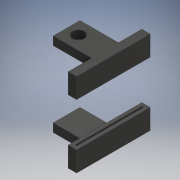
# Autodesk Inventor part: learnbotAgarreCamara
Saved by Autodesk Inventor 2017 (Build 210142000, 142)
## iProperties
Part Number: learnbotAgarreCamara
Material: Genérico
Document SubType Name: Modeling
Designer: rober
Density: 1 g/cm^3
Appearance: Valor por defecto
Author: rober
Autodesk Inventor part; units mm, degrees
ref_plane "YZ Plane" through (0, 0, 0) normal (1, 0, 0) x (0, 1, 0)
ref_plane "XZ Plane" through (0, 0, 0) normal (0, 1, 0) x (-1, 0, 0)
ref_plane "XY Plane" through (0, 0, 0) normal (0, 0, 1) x (1, 0, 0)
sketch "Boceto8" plane through (0, 0, 0) normal (0, 0, 1) x (1, 0, 0)
  line L0 (-2.8, 3) -> (-0.5, 3)
  line L1 (-0.5, 1.4) -> (-2.8, 1.4)
  line L2 (-2.8, 3) -> (-2.8, 1.4)
  line L3 (0, 3) -> (0, 0)
  line L4 (0, 0) -> (-0.5, 0)
  line L5 (-0.5, 0) -> (-0.5, 1.4)
  line L6 (0, 3) -> (0, 4.4)
  line L7 (0, 4.4) -> (-0.5, 4.4)
  line L8 (-0.5, 4.4) -> (-0.5, 3)
  constraints: 18 end point
extrude "Extrusión8" add sketch "Boceto8" along normal blind 0.5
sketch "Boceto9" plane through (0, 0, 0.5) normal (0, 0, 1) x (1, 0, 0)
  line L0 (-0.5, 3) -> (-2.8, 3) projected
  line L1 (-2.8, 3) -> (-2.8, 1.4) projected
  line L2 (-2.8, 1.4) -> (-0.5, 1.4) projected
  line L3 (-0.5, 1.4) -> (-0.5, 0) projected
  line L4 (-0.5, 0) -> (0, 0) projected
  line L5 (0, 0) -> (0, 4.4) projected
  line L6 (0, 4.4) -> (-0.5, 4.4) projected
  line L7 (-0.5, 4.4) -> (-0.5, 3) projected
  line L8 (0, 4.4) -> (0, 0) projected
  line L9 (-0.5, 4.4) -> (0, 4.4)
  line L10 (0, 4.4) -> (0, 0)
  line L11 (0, 0) -> (-0.5, 0)
  line L12 (-0.5, 0) -> (-0.5, 4.4)
  constraints: 8 end point, 2 parallel, 1 horizontal, 1 perpendicular
extrude "Extrusión9" add sketch "Boceto9" along normal blind 0.7 contours L7 L6 L5 L4 L3 L12
sketch "Boceto10" plane through (0, 0, 0) normal (0, 0, -1) x (-1, 0, 0)
  line L0 (2.8, 3) -> (0.5, 3)
  line L1 (0.5, 3) -> (0.5, 4.4)
  line L2 (0.5, 4.4) -> (0, 4.4)
  line L3 (0, 4.4) -> (0, 0)
  line L4 (0, 0) -> (0.5, 0)
  line L5 (0.5, 0) -> (0.5, 1.4)
  line L6 (0.5, 1.4) -> (2.8, 1.4)
  line L7 (2.8, 1.4) -> (2.8, 3)
  arc A0 (1.893104, 1.910428) -> (1.925936, 2.512803) centre (2.122635, 2.2) ccw
  line L8 (0.685113, 2.000554) -> (1.893104, 1.910428)
  line L9 (0.681802, 2.399171) -> (1.925936, 2.512803)
  arc A1 (0.681802, 2.399171) -> (0.685113, 2.000554) centre (0.699993, 2.2) ccw
  line L10 (2.8, 1.4) -> (0.499993, 1.4)
  line L11 (0.499993, 3) -> (2.8, 3)
  line L12 (2.8, 1.4) -> (2.8, 3)
  line L13 (-0.000007, 1.4) -> (-0.000007, 4.4)
  line L14 (-0.000007, 4.4) -> (0.499993, 4.4)
  line L15 (0.499993, 4.4) -> (0.499993, 3)
  line L16 (-0.000007, 1.4) -> (-0.000007, 0)
  line L17 (-0.000007, 0) -> (0.499993, 0)
  line L18 (0.499993, 0) -> (0.499993, 1.4)
  line L19 (0.299993, 1.4) -> (0.299993, 4.2)
  line L20 (0.299993, 4.2) -> (0.199993, 4.2)
  line L21 (0.199993, 4.2) -> (0.199993, 1.4)
  line L22 (0.299993, 1.4) -> (0.299993, 0.2)
  line L23 (0.299993, 0.2) -> (0.199993, 0.2)
  line L24 (0.199993, 0.2) -> (0.199993, 1.4)
  line L25 (0.499993, 1.4) -> (0.499993, 3)
  constraints: 36 end point, 4 point on circle, 2 centre point
sketch "Boceto10 outline for Extrusión10" plane through (0, 0, 0) normal (0, 0, -1) x (-1, 0, 0)
  line L0 (0.685113, 2.000554) -> (1.893104, 1.910428)
  arc A0 (0.681802, 2.399171) -> (0.685113, 2.000554) centre (0.699993, 2.2) ccw
  line L1 (1.925936, 2.512803) -> (0.681802, 2.399171)
  arc A1 (1.893104, 1.910428) -> (1.925936, 2.512803) centre (2.122635, 2.2) ccw
extrude "Extrusión10" cut sketch "Boceto10 outline for Extrusión10" against normal blind 0.25
sketch "Boceto11" plane through (0, 0, 1.2) normal (0, 0, 1) x (1, 0, 0)
  line L0 (0, 0) -> (0, 4.4)
  line L1 (0, 4.4) -> (-0.5, 4.4)
  line L2 (-0.5, 4.4) -> (-0.5, 0)
  line L3 (-0.5, 0) -> (0, 0)
  arc A0 (-1.893111, 2.489572) -> (-1.925943, 1.887197) centre (-2.122641, 2.2) ccw
  line L4 (-0.68512, 2.399446) -> (-1.893111, 2.489572)
  line L5 (-0.681809, 2.000829) -> (-1.925943, 1.887197)
  arc A1 (-0.681809, 2.000829) -> (-0.68512, 2.399446) centre (-0.7, 2.2) ccw
  line L6 (-2.800007, 3) -> (-0.5, 3)
  line L7 (-0.5, 1.4) -> (-2.800007, 1.4)
  line L8 (-2.800007, 3) -> (-2.800007, 1.4)
  line L9 (0, 3) -> (0, 0)
  line L10 (0, 0) -> (-0.5, 0)
  line L11 (-0.5, 0) -> (-0.5, 1.4)
  line L12 (0, 3) -> (0, 4.4)
  line L13 (0, 4.4) -> (-0.5, 4.4)
  line L14 (-0.5, 4.4) -> (-0.5, 3)
  line L15 (-0.3, 3) -> (-0.3, 0.2)
  line L16 (-0.3, 0.2) -> (-0.2, 0.2)
  line L17 (-0.2, 0.2) -> (-0.2, 3)
  line L18 (-0.3, 3) -> (-0.3, 4.2)
  line L19 (-0.3, 4.2) -> (-0.2, 4.2)
  line L20 (-0.2, 4.2) -> (-0.2, 3)
  line L21 (-0.5, 3) -> (-0.5, 1.4)
  constraints: 36 end point, 4 point on circle, 2 centre point
extrude "Extrusión11" cut sketch "Boceto11" against normal blind 0.7 contours L18 L19 L20 L17 L16 L15
sketch "Boceto12" plane through (0, 0, 0) normal (1, 0, 0) x (0, 0, -1)
  line L0 (-5, 4.4) -> (-3.8, 4.4)
  line L1 (-3.8, 0) -> (-5, 0)
  line L2 (-5, 0) -> (-5, 4.4)
  line L3 (-5, 4.4) -> (-3.8, 4.4)
  line L4 (-3.8, 4.4) -> (-3.8, 0)
  point P0 (-0.5, 0.2)
  point P1 (0, 4.4)
  constraints: 10 end point
extrude "Extrusión12" add sketch "Boceto12" against normal blind 0.5
sketch "Boceto13" plane through (-0.5, 0, 0) normal (-1, 0, 0) x (0, 0, 1)
  line L0 (0, 1.4) -> (0, 3) projected
  line L1 (0, 1.4) -> (0.5, 1.4) projected
  line L2 (0.5, 3) -> (0.5, 1.4) projected
  line L3 (0, 3) -> (0.5, 3) projected
  line L4 (0, 3) -> (0.5, 3)
  line L5 (0.5, 3) -> (0.5, 1.4)
  line L6 (0.5, 1.4) -> (0, 1.4)
  line L7 (0, 1.4) -> (0, 3)
  line L8 (4.5, 3) -> (5, 3)
  line L9 (5, 3) -> (5, 1.4)
  line L10 (5, 1.4) -> (4.5, 1.4)
  line L11 (4.5, 1.4) -> (4.5, 3)
  point P0 (0, 0)
  constraints: 16 end point, 4 parallel, 2 horizontal, 2 perpendicular
extrude "Extrusión13" add sketch "Boceto13" along normal blind 2.3 contours L8 L9 L10 L11
sketch "Boceto14" plane through (0, 0, 3.8) normal (0, 0, -1) x (-1, 0, 0)
  line L0 (0.2, 4.2) -> (0.2, 0.2) projected
  line L1 (0.3, 0.2) -> (0.3, 4.2) projected
  line L2 (0.2, 4.2) -> (0.3, 4.2)
  line L3 (0.3, 4.2) -> (0.3, 0.2)
  line L4 (0.3, 0.2) -> (0.2, 0.2)
  line L5 (0.2, 0.2) -> (0.2, 4.2)
  point P0 (0, 0)
  constraints: 8 end point, 2 parallel, 1 horizontal, 1 perpendicular
extrude "Extrusión14" cut sketch "Boceto14" against normal blind 0.7
sketch "Boceto15" plane through (0, 0, 5) normal (0, 0, 1) x (1, 0, 0)
  circle A0 centre (-2.1, 2.2) radius 0.369508
  line L0 (-2.8, 3) -> (-0.5, 3)
  line L1 (-0.5, 1.4) -> (-2.8, 1.4)
  line L2 (-2.8, 3) -> (-2.8, 1.4)
  line L3 (0, 3) -> (0, 0)
  line L4 (0, 0) -> (-0.5, 0)
  line L5 (-0.5, 0) -> (-0.5, 1.4)
  line L6 (0, 3) -> (0, 4.4)
  line L7 (0, 4.4) -> (-0.5, 4.4)
  line L8 (-0.5, 4.4) -> (-0.5, 3)
  line L9 (0, 4.4) -> (0, 0)
  line L10 (0, 4.4) -> (-0.5, 4.4)
  line L11 (-0.5, 3) -> (-0.5, 4.4)
  line L12 (-0.5, 3) -> (-2.8, 3)
  line L13 (-2.8, 1.4) -> (-2.8, 3)
  line L14 (-0.5, 1.4) -> (-2.8, 1.4)
  line L15 (-0.5, 0) -> (-0.5, 1.4)
  line L16 (0, 0) -> (-0.5, 0)
  constraints: 18 end point, 1 centre point
extrude "Extrusión15" cut sketch "Boceto15" against normal blind 0.9 contours A0
